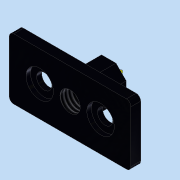
# Autodesk Inventor part: Metric 8mm ACME Nut Plate
Saved by Autodesk Inventor 2013 SP2 (Build 170200200, 200)
## iProperties
Created: 2014-04-23
Part Number: Metric 8mm ACME Nut Plate
Material: Acetal Resin, Black
Document SubType Name: Modeling
Designer: Work
Density: 1.425 g/cm^3
Catalog Web Link: www.openbuilds.org
Vendor: OpenBuilds
Mass: 4.1221 g
Surface Area: 25.8878 cm^2
Volume: 2.89271 cm^3
Author: Work
Autodesk Inventor part; units mm, degrees
ref_plane "YZ Plane" through (0, 0, 0) normal (1, 0, 0) x (0, 1, 0)
ref_plane "XZ Plane" through (0, 0, 0) normal (0, 1, 0) x (-1, 0, 0)
ref_plane "XY Plane" through (0, 0, 0) normal (0, 0, 1) x (1, 0, 0)
sketch "Sketch1" plane through (0, 0, 0) normal (0, 1, 0) x (-1, 0, 0)
  line L0 (20, -10) -> (-20, -10)
  line L1 (-20, -10) -> (-20, 10)
  line L2 (-20, 10) -> (20, 10)
  line L3 (20, 10) -> (20, -10)
  line L4 (20, -10) -> (-20, 10) construction
  line L5 (-20, -10) -> (20, 10) construction
  point P0 (0, 0)
  dimension "d0" = 40
  dimension "d1" = 20
  constraints: 12 end point, 2 midpoint, 2 parallel, 1 horizontal, 1 perpendicular
  measures "d0" distance of L1.end L2.end
  measures "d1" distance of L0.end L1.end
extrude "Extrusion1" add sketch "Sketch1" along normal blind 3.2
sketch "Sketch2" plane through (0, 0, 0) normal (0, -1, 0) x (1, 0, 0)
  line L0 (-20, -10) -> (20, -10) projected
  line L1 (-20, 10) -> (-20, -10) projected
  point P0 (0, 0)
  point P1 (-10, 0)
  point P2 (10, 0)
  dimension "d4" = 10
  dimension "d5" = 20
  dimension "d6" = 10
  constraints: 1 horizontal alignment
  measures "d4" distance from line of point (-10, 0) L1
  measures "d5" distance of point (10, 0) point (-10, 0)
  measures "d6" distance from line of L0 point (-10, 0)
hole "Hole1" at (-10, 0, 0) at (10, 0, 0) direction (0, 1, 0) diameter 5 end through all counterbore diameter 9 counterbore depth 1.5
sketch "Sketch3" plane through (0, 3.2, 0) normal (0, 1, 0) x (1, 0, 0)
  line L0 (-20, -10) -> (20, -10) projected
  line L1 (2.3776, -5.74) -> (-2.3776, -5.74)
  line L2 (-2.3776, -5.74) -> (-5.74, -2.3776)
  line L3 (-5.74, -2.3776) -> (-5.74, 2.3776)
  line L4 (-5.74, 2.3776) -> (-2.3776, 5.74)
  line L5 (-2.3776, 5.74) -> (2.3776, 5.74)
  line L6 (2.3776, 5.74) -> (5.74, 2.3776)
  line L7 (5.74, 2.3776) -> (5.74, -2.3776)
  line L8 (5.74, -2.3776) -> (2.3776, -5.74)
  point P0 (0, 0)
  point P1 (0, 0)
  dimension "d14" = 11.48
  constraints: 16 end point, 1 coincident, 1 parallel, 17 other
  measures "d14" distance between parallel lines of L5 L1
extrude "Extrusion2" add sketch "Sketch3" along normal blind 9.5
sketch "Sketch4" plane through (0, 12.7, 0) normal (0, 1, 0) x (1, 0, 0)
  point P0 (0, 0)
  point P1 (0, 0)
  constraints: 1 coincident
hole "Hole2" at (0, 12.7, 0) direction (0, -1, 0) diameter 6.647 end through all thread size "M8x1.25" class "6H" standard "ANSI Metric M Profile"
fillet "Fillet1" radius 1.5 4 edges at (-20, 1.6, 10) (20, 1.6, 10) (20, 1.6, -10) (-20, 1.6, -10)
body "Solid1"
